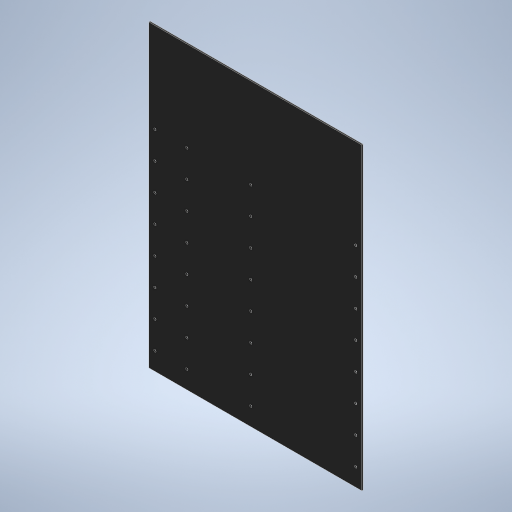
# Autodesk Inventor part: Side Panel
Saved by Autodesk Inventor 2024 (Build 280153000, 153)
## iProperties
Created: 2024-08-28
Part Number: Side Panel
Material: PET Plastic
Document SubType Name: Modeling
Designer: Ishaan
Density: 1.541 g/cm^3
Appearance: Polycarbonate - Clear
Author: Ishaan
Autodesk Inventor part; units mm, degrees
ref_plane "YZ Plane" through (0, 0, 0) normal (1, 0, 0) x (0, 1, 0)
ref_plane "XZ Plane" through (0, 0, 0) normal (0, 1, 0) x (-1, 0, 0)
ref_plane "XY Plane" through (0, 0, 0) normal (0, 0, 1) x (1, 0, 0)
sketch "Sketch1" plane through (0, 0, 0) normal (0, 0, 1) x (1, 0, 0)
  line L0 (233.35, -328) -> (-233.35, -328)
  line L1 (-233.35, -328) -> (-233.35, 328)
  line L2 (-233.35, 328) -> (233.35, 328)
  line L3 (233.35, 328) -> (233.35, -328)
  line L4 (233.35, -328) -> (-233.35, 328) construction
  line L5 (-233.35, -328) -> (233.35, 328) construction
  point P0 (0, 0)
  dimension "d0" = 466.7
  dimension "d1" = 656
  constraints: 12 end point, 2 midpoint, 2 parallel, 1 horizontal, 1 perpendicular
  measures "d0" distance of L1.end L2.end
  measures "d1" distance of L0.end L1.end
extrude "Extrusion1" add sketch "Sketch1" along normal mid plane 3
sketch "Sketch2" plane through (0, 0, -1.5) normal (0, 0, -1) x (-1, 0, 0)
  line L0 (220, -289) -> (-220, -289) construction
  line L1 (-220, -289) -> (-220, 191) construction
  line L2 (-220, 191) -> (220, 191) construction
  line L3 (220, 191) -> (220, -289) construction
  line L4 (220, -289) -> (-220, 191) construction
  line L5 (-220, -289) -> (220, 191) construction
  line L6 (-233.35, -328) -> (233.35, -328) construction
  line L7 (150, -289) -> (150, 191) construction
  line L8 (10, -289) -> (10, 191) construction
  point P0 (0, 0)
  point P1 (0, -49)
  point P2 (-220, -229)
  point P3 (10, -229)
  point P4 (150, -229)
  point P5 (220, -229)
  point P6 (-220, -169)
  point P7 (10, -169)
  point P8 (150, -169)
  point P9 (220, -169)
  point P10 (-220, -109)
  point P11 (10, -109)
  point P12 (150, -109)
  point P13 (220, -109)
  point P14 (-220, -49)
  point P15 (10, -49)
  point P16 (150, -49)
  point P17 (220, -49)
  point P18 (-220, 11)
  point P19 (10, 11)
  point P20 (150, 11)
  point P21 (220, 11)
  point P22 (-220, 71)
  point P23 (10, 71)
  point P24 (150, 71)
  point P25 (220, 71)
  point P26 (-220, 131)
  point P27 (10, 131)
  point P28 (150, 131)
  point P29 (220, 131)
  dimension "d8" = 440
  dimension "d9" = 39
  dimension "d25" = 480
  dimension "d26" = 70
  dimension "d27" = 210
  dimension "d30" = 60
  constraints: 16 end point, 4 coincident, 4 point on line, 2 midpoint, 2 parallel, 2 perpendicular, 2 vertical, 1 horizontal, 1 vertical alignment, 28 other
  measures "d8" distance of L1.end L2.end
  measures "d9" distance between parallel lines of L6 L0
  measures "d25" distance of L2.end L0.start
  measures "d26" distance between parallel lines of L3 L7
  measures "d27" distance between parallel lines of L3 L8
  measures "d30" distance of point (-220, -289) point (-220, -229)
hole "Hole2" at (220, -289, -1.5) at (-220, -289, -1.5) at (-10, -289, -1.5) at (-150, -289, -1.5) at (220, -229, -1.5) at (-10, -229, -1.5) at (-150, -229, -1.5) at (-220, -229, -1.5) at (220, -169, -1.5) at (-10, -169, -1.5) at (-150, -169, -1.5) at (-220, -169, -1.5) at (220, -109, -1.5) at (-10, -109, -1.5) at (-150, -109, -1.5) at (-220, -109, -1.5) at (220, -49, -1.5) at (-10, -49, -1.5) at (-150, -49, -1.5) at (-220, -49, -1.5) at (220, 11, -1.5) at (-10, 11, -1.5) at (-150, 11, -1.5) at (-220, 11, -1.5) at (220, 71, -1.5) at (-10, 71, -1.5) at (-150, 71, -1.5) at (-220, 71, -1.5) at (220, 131, -1.5) at (-10, 131, -1.5) at (-150, 131, -1.5) at (-220, 131, -1.5) direction (0, 0, 1) diameter 5.3 end through all
